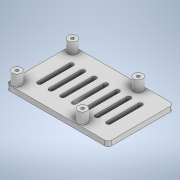
# Autodesk Inventor part: Base Rev A
Saved by Autodesk Inventor 2021 (Build 250183000, 183)
## iProperties
Created: 2020-10-18
Part Number: Base Rev A
Material: Generic
Document SubType Name: Modeling
Designer: cmzgt
Density: 1 g/cm^3
Appearance: Default
Author: cmzgt
## iProperties of the stored document _3DPrint.ipt
Created: 2020-10-18
Part Number: _3DPrint
Material: Generic
Document SubType Name: Modeling
Designer: cmzgt
Density: 1 g/cm^3
Appearance: Default
Author: cmzgt
Autodesk Inventor part; units mm, degrees
ref_plane "YZ Plane" through (0, 0, 0) normal (1, 0, 0) x (0, 1, 0)
ref_plane "XZ Plane" through (0, 0, 0) normal (0, 1, 0) x (-1, 0, 0)
ref_plane "XY Plane" through (0, 0, 0) normal (0, 0, 1) x (1, 0, 0)
sketch "Sketch1" plane through (0, 0, 0) normal (0, 1, 0) x (-1, 0, 0)
  line L0 (-45, -29) -> (45, -29)
  line L1 (45, -29) -> (45, 29)
  line L2 (45, 29) -> (-45, 29)
  line L3 (-45, 29) -> (-45, -29)
  line L4 (-45, -29) -> (45, 29) construction
  line L5 (45, -29) -> (-45, 29) construction
  point P0 (0, 0)
  dimension "d0" = 90
  dimension "d1" = 58
  constraints: 12 end point, 2 midpoint, 2 parallel, 1 horizontal, 1 perpendicular
  measures "d0" distance of L2.end L1.end
  measures "d1" distance of L1.end L0.end
extrude "Extrusion1" add sketch "Sketch1" along normal blind 4.445
fillet "Fillet2" radius 3 4 edges at (45, 2.2225, 29) (-45, 2.2225, 29) (45, 2.2225, -29) (-45, 2.2225, -29)
sketch "Sketch4" plane through (0, 4.445, 0) normal (0, 1, 0) x (1, 0, 0)
  line L0 (0, -13.97) -> (0, 13.97) construction
  line L1 (1.905, -13.97) -> (1.905, 13.97)
  line L2 (-1.905, 13.97) -> (-1.905, -13.97)
  arc A0 (-1.905, -13.97) -> (1.905, -13.97) centre (0, -13.97) ccw
  arc A1 (1.905, 13.97) -> (-1.905, 13.97) centre (0, 13.97) ccw
  line L3 (42, 29) -> (-42, 29) construction
  line L4 (0, 29) -> (0, -29) construction
  line L5 (-42, -29) -> (42, -29) construction
  line L6 (45, -26) -> (45, 26) construction
  line L7 (45, 0) -> (-45, 0) construction
  line L8 (-45, 26) -> (-45, -26) construction
  line L9 (-8.255, -13.97) -> (-8.255, 13.97)
  line L10 (-12.065, 13.97) -> (-12.065, -13.97)
  arc A2 (-8.255, 13.97) -> (-12.065, 13.97) centre (-10.16, 13.97) ccw
  arc A3 (-12.065, -13.97) -> (-8.255, -13.97) centre (-10.16, -13.97) ccw
  line L11 (-18.415, -13.97) -> (-18.415, 13.97)
  line L12 (-22.225, 13.97) -> (-22.225, -13.97)
  arc A4 (-18.415, 13.97) -> (-22.225, 13.97) centre (-20.32, 13.97) ccw
  arc A5 (-22.225, -13.97) -> (-18.415, -13.97) centre (-20.32, -13.97) ccw
  line L13 (-28.575, -13.97) -> (-28.575, 13.97)
  line L14 (-32.385, 13.97) -> (-32.385, -13.97)
  arc A6 (-28.575, 13.97) -> (-32.385, 13.97) centre (-30.48, 13.97) ccw
  arc A7 (-32.385, -13.97) -> (-28.575, -13.97) centre (-30.48, -13.97) ccw
  line L15 (12.065, -13.97) -> (12.065, 13.97)
  line L16 (8.255, 13.97) -> (8.255, -13.97)
  arc A8 (12.065, 13.97) -> (8.255, 13.97) centre (10.16, 13.97) ccw
  arc A9 (8.255, -13.97) -> (12.065, -13.97) centre (10.16, -13.97) ccw
  line L17 (1.905, -13.97) -> (1.905, 13.97)
  line L18 (-1.905, 13.97) -> (-1.905, -13.97)
  arc A10 (1.905, 13.97) -> (-1.905, 13.97) centre (0, 13.97) ccw
  arc A11 (-1.905, -13.97) -> (1.905, -13.97) centre (0, -13.97) ccw
  line L19 (-8.255, -13.97) -> (-8.255, 13.97)
  line L20 (-12.065, 13.97) -> (-12.065, -13.97)
  arc A12 (-8.255, 13.97) -> (-12.065, 13.97) centre (-10.16, 13.97) ccw
  arc A13 (-12.065, -13.97) -> (-8.255, -13.97) centre (-10.16, -13.97) ccw
  line L21 (-18.415, -13.97) -> (-18.415, 13.97)
  line L22 (-22.225, 13.97) -> (-22.225, -13.97)
  arc A14 (-18.415, 13.97) -> (-22.225, 13.97) centre (-20.32, 13.97) ccw
  arc A15 (-22.225, -13.97) -> (-18.415, -13.97) centre (-20.32, -13.97) ccw
  line L23 (22.225, -13.97) -> (22.225, 13.97)
  line L24 (18.415, 13.97) -> (18.415, -13.97)
  arc A16 (22.225, 13.97) -> (18.415, 13.97) centre (20.32, 13.97) ccw
  arc A17 (18.415, -13.97) -> (22.225, -13.97) centre (20.32, -13.97) ccw
  line L25 (12.065, -13.97) -> (12.065, 13.97)
  line L26 (8.255, 13.97) -> (8.255, -13.97)
  arc A18 (12.065, 13.97) -> (8.255, 13.97) centre (10.16, 13.97) ccw
  arc A19 (8.255, -13.97) -> (12.065, -13.97) centre (10.16, -13.97) ccw
  line L27 (1.905, -13.97) -> (1.905, 13.97)
  line L28 (-1.905, 13.97) -> (-1.905, -13.97)
  arc A20 (1.905, 13.97) -> (-1.905, 13.97) centre (0, 13.97) ccw
  arc A21 (-1.905, -13.97) -> (1.905, -13.97) centre (0, -13.97) ccw
  line L29 (-8.255, -13.97) -> (-8.255, 13.97)
  line L30 (-12.065, 13.97) -> (-12.065, -13.97)
  arc A22 (-8.255, 13.97) -> (-12.065, 13.97) centre (-10.16, 13.97) ccw
  arc A23 (-12.065, -13.97) -> (-8.255, -13.97) centre (-10.16, -13.97) ccw
  line L31 (32.385, -13.97) -> (32.385, 13.97)
  line L32 (28.575, 13.97) -> (28.575, -13.97)
  arc A24 (32.385, 13.97) -> (28.575, 13.97) centre (30.48, 13.97) ccw
  arc A25 (28.575, -13.97) -> (32.385, -13.97) centre (30.48, -13.97) ccw
  line L33 (22.225, -13.97) -> (22.225, 13.97)
  line L34 (18.415, 13.97) -> (18.415, -13.97)
  arc A26 (22.225, 13.97) -> (18.415, 13.97) centre (20.32, 13.97) ccw
  arc A27 (18.415, -13.97) -> (22.225, -13.97) centre (20.32, -13.97) ccw
  line L35 (12.065, -13.97) -> (12.065, 13.97)
  line L36 (8.255, 13.97) -> (8.255, -13.97)
  arc A28 (12.065, 13.97) -> (8.255, 13.97) centre (10.16, 13.97) ccw
  arc A29 (8.255, -13.97) -> (12.065, -13.97) centre (10.16, -13.97) ccw
  line L37 (1.905, -13.97) -> (1.905, 13.97)
  line L38 (-1.905, 13.97) -> (-1.905, -13.97)
  arc A30 (1.905, 13.97) -> (-1.905, 13.97) centre (0, 13.97) ccw
  arc A31 (-1.905, -13.97) -> (1.905, -13.97) centre (0, -13.97) ccw
  point P0 (0, 0)
  dimension "d18" = 13.97
  dimension "d19" = 3.81
  dimension "d22" = 10.16
  dimension "d25" = 10.16
  constraints: 72 end point, 64 point on circle, 32 centre point, 5 midpoint, 4 tangent, 2 horizontal, 1 parallel, 1 vertical, 150 other
  measures "d18" distance of point (0, 0) L0.end
  measures "d19" diameter of A1
  measures "d22" distance of L1.start L9.start
  measures "d25" distance of L1.start L15.start
extrude "Extrusion3" cut sketch "Sketch4" against normal blind 4.445
sketch "Sketch5" plane through (0, 4.445, 0) normal (0, 1, 0) x (1, 0, 0)
  circle A0 centre (-40, 24.5) radius 4
  circle A1 centre (-40, 24.5) radius 1.375
  line L0 (-45, 26) -> (-45, -26) projected
  line L1 (42, 29) -> (-42, 29) projected
  line L2 (-45, 0) -> (45, 0)
  line L3 (45, -26) -> (45, 26) projected
  circle A2 centre (-40, -24.5) radius 4
  circle A3 centre (-40, -24.5) radius 1.375
  circle A4 centre (18, 24.5) radius 4
  circle A5 centre (18, 24.5) radius 1.375
  circle A6 centre (18, -24.5) radius 4
  circle A7 centre (18, -24.5) radius 1.375
  line L4 (-42, -29) -> (42, -29) projected
  point P0 (0, 0)
  dimension "d35" = 8
  dimension "d36" = 2.75
  dimension "d37" = 5
  dimension "d39" = 8
  dimension "d40" = 2.75
  dimension "d41" = 58
  dimension "d43" = 4.5
  dimension "d45" = 8
  dimension "d46" = 2.75
  dimension "d47" = 49
  dimension "d50" = 58
  dimension "d51" = 4.5
  constraints: 8 centre point, 4 coincident, 2 end point, 2 midpoint, 2 symmetric about line, 2 other
  measures "d35" diameter of A0
  measures "d36" diameter of A1
  measures "d37" distance from line of L0 A0.centre
  measures "d39" diameter of A4
  measures "d40" diameter of A5
  measures "d41" distance of A1.centre A5.centre
  measures "d43" distance from line of L1 A4.centre
  measures "d45" diameter of A6
  measures "d46" diameter of A7
  measures "d47" distance of A0.centre A2.centre
  measures "d50" distance of A2.centre A7.centre
  measures "d51" distance from line of L4 A6.centre
extrude "Extrusion4" add sketch "Sketch5" along normal blind 10
body "Solid1"
